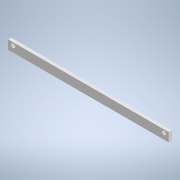
# Autodesk Inventor part: Carcasa_Tope
Saved by Autodesk Inventor 2022 (Build 260153000, 153)
## iProperties
Created: 2022-02-22
Part Number: Carcasa_Tope
Material: Generic
Document SubType Name: Modeling
Designer: katha
Density: 1 g/cm^3
Appearance: Default
Author: katha
Autodesk Inventor part; units mm, degrees
ref_plane "YZ Plane" through (0, 0, 0) normal (1, 0, 0) x (0, 1, 0)
ref_plane "XZ Plane" through (0, 0, 0) normal (0, 1, 0) x (-1, 0, 0)
ref_plane "XY Plane" through (0, 0, 0) normal (0, 0, 1) x (1, 0, 0)
sketch "Sketch1" plane through (0, 0, 0) normal (0, 0, 1) x (1, 0, 0)
  circle A0 centre (-76, 12) radius 2 projected
  circle A1 centre (76, 12) radius 2 projected
  line L0 (-81, 15.7) -> (81, 15.7)
  line L1 (81, 15.7) -> (81, 6.7)
  line L2 (81, 6.7) -> (-81, 6.7)
  line L3 (-81, 6.7) -> (-81, 15.7)
  line L4 (-85, 20) -> (-85, -20) projected
  line L5 (85, -20) -> (85, 20) projected
  line L6 (-44.0994, 17.1019) -> (-47.4458, 17.1019) projected
  line L7 (-42.4262, 20) -> (-44.0994, 17.1019) projected
  line L8 (-44.0994, 22.8981) -> (-42.4262, 20) projected
  line L9 (-47.4458, 22.8981) -> (-44.0994, 22.8981) projected
  line L10 (-49.119, 20) -> (-47.4458, 22.8981) projected
  line L11 (-47.4458, 17.1019) -> (-49.119, 20) projected
  line L12 (-53.5726, 20) -> (-85, 20) projected
  line L13 (-48.6707, 21.6732) -> (-42.8745, 18.3268)
  line L14 (-45.7726, 23.3464) -> (-45.7726, 16.6536)
  line L15 (-42.8745, 21.6732) -> (-48.6707, 18.3268)
  line L16 (-45.7726, 20) -> (-45.7726, 21.9321)
  point P0 (0, 0)
  dimension "d0" = 162
  dimension "d1" = 9
  dimension "d2" = 4
  dimension "d3" = 3.7
  constraints: 16 end point, 2 parallel, 1 horizontal, 1 perpendicular, 1 vertical
  measures "d0" distance of L1.end L2.end
  measures "d1" distance of L0.end L1.end
  measures "d2" distance between parallel lines of L4 L3
  measures "d3" distance from line of A0.centre L0
extrude "Extrusion1" add sketch "Sketch1" along normal blind 3.2 contours L0 L1 L2 L3
body "Solid1"
